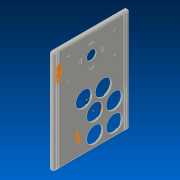
# Autodesk Inventor part: Top
Saved by Autodesk Inventor 2016 (Build 200138000, 138)
## iProperties
Created: 2015-08-21
Part Number: Top
Material: Generic
Document SubType Name: Modeling
Designer: Moffitt
Density: 1 g/cm^3
Appearance: Default
Author: Moffitt
Autodesk Inventor part; units mm, degrees
ref_plane "YZ Plane" through (0, 0, 0) normal (1, 0, 0) x (0, 1, 0)
ref_plane "XZ Plane" through (0, 0, 0) normal (0, 1, 0) x (-1, 0, 0)
ref_plane "XY Plane" through (0, 0, 0) normal (0, 0, 1) x (1, 0, 0)
sketch "Top-Body" plane through (0, 0, 0) normal (1, 0, 0) x (0, 1, 0)
  line L0 (107.2007, 64.0864) -> (-82.7993, 64.0864)
  line L1 (-82.7993, 64.0864) -> (-82.7993, -75.9136)
  line L2 (-82.7993, -75.9136) -> (107.2007, -75.9136)
  line L3 (107.2007, -75.9136) -> (107.2007, 64.0864)
  circle A0 centre (69.2007, -5.9136) radius 9
  circle A1 centre (6.2007, -27.9136) radius 15
  circle A2 centre (-24.2993, -47.9136) radius 15
  circle A3 centre (-60.2993, -47.9136) radius 15
  circle A4 centre (6.2007, 8.0864) radius 15
  circle A5 centre (-24.2993, -11.9136) radius 15
  circle A6 centre (-60.2993, -11.9136) radius 15
  circle A7 centre (89.2007, 36.0864) radius 2.5
  circle A8 centre (89.2007, -47.9136) radius 2.5
  circle A9 centre (49.2007, -47.9136) radius 2.5
  circle A10 centre (49.2007, 36.0864) radius 2.5
  point P0 (0, 0)
  dimension "d0" = 190
  dimension "d1" = 140
  dimension "d2" = 18
  dimension "d3" = 38
  dimension "d5" = 30
  dimension "d6" = 30
  dimension "d7" = 20
  dimension "d8" = 30.5
  dimension "d9" = 30
  dimension "d10" = 36
  dimension "d11" = 0
  dimension "d12" = 63
  dimension "d13" = 30
  dimension "d14" = 30
  dimension "d15" = 30
  dimension "d16" = 36
  dimension "d17" = 36
  dimension "d18" = 36
  dimension "d19" = 0
  dimension "d20" = 0
  dimension "d21" = 0
  dimension "d23" = 14
  dimension "d24" = 70
  dimension "d25" = 5
  dimension "d26" = 42
  dimension "d27" = 20
  dimension "d28" = 20
  dimension "d29" = 20
  dimension "d30" = 20
  dimension "d31" = 42
  dimension "d32" = 42
  dimension "d33" = 70
  dimension "d146" = 42
  dimension "d149" = 5
  dimension "d150" = 5
  dimension "d151" = 5
  constraints: 11 centre point, 8 end point, 2 parallel, 1 horizontal, 1 perpendicular
  measures "d0" distance of L0.start L0.end
  measures "d1" distance of L2.end L0.start
  measures "d2" diameter of A0
  measures "d3" distance from line of L3 A0.centre
  measures "d5" diameter of A1
  measures "d6" diameter of A2
  measures "d7" vertical distance of A2.centre A1.centre
  measures "d8" horizontal distance of A2.centre A1.centre
  measures "d9" diameter of A3
  measures "d10" distance of A3.centre A2.centre
  measures "d11" vertical distance of A3.centre A2.centre
  measures "d12" horizontal distance of A1.centre A0.centre
  measures "d13" diameter of A4
  measures "d14" diameter of A5
  measures "d15" diameter of A6
  measures "d16" distance of A1.centre A4.centre
  measures "d17" distance of A2.centre A5.centre
  measures "d18" distance of A3.centre A6.centre
  measures "d19" horizontal distance of A4.centre A1.centre
  measures "d20" horizontal distance of A5.centre A2.centre
  measures "d21" horizontal distance of A6.centre A3.centre
  measures "d23" vertical distance of A0.centre A4.centre
  measures "d24" distance from line of L2 A0.centre
  measures "d25" diameter of A7
  measures "d26" vertical distance of A0.centre A7.centre
  measures "d27" horizontal distance of A7.centre A0.centre
  measures "d28" horizontal distance of A10.centre A0.centre
  measures "d29" horizontal distance of A0.centre A8.centre
  measures "d30" horizontal distance of A9.centre A0.centre
  measures "d31" vertical distance of A0.centre A8.centre
  measures "d32" vertical distance of A9.centre A0.centre
  measures "d33" distance from line of L0 A0.centre
  measures "d146" vertical distance of A0.centre A10.centre
  measures "d149" diameter of A10
  measures "d150" diameter of A9
  measures "d151" diameter of A8
extrude "Main Face" add sketch "Top-Body" along normal blind 3
fillet "Top Fillet" radius 3 4 edges at (3, 107.2007, -5.9136) (3, 12.2007, 64.0864) (3, 12.2007, -75.9136) (3, -82.7993, -5.9136)
sketch "Button clip cutouts" plane through (0, 0, 0) normal (-1, 0, 0) x (0, 0, 1)
  line L0 (-33.0644, -51.1069) -> (-38.7212, -45.45)
  line L1 (-38.7212, -45.45) -> (-63.7628, -70.4917)
  line L2 (-63.7628, -70.4917) -> (-58.106, -76.1485)
  line L3 (-58.106, -76.1485) -> (-33.0644, -51.1069)
  line L4 (64.0864, -82.7993) -> (-75.9136, -82.7993) projected
  line L5 (3.9356, -70.4917) -> (-1.7212, -76.1485)
  line L6 (-1.7212, -76.1485) -> (-26.7628, -51.1069)
  line L7 (-26.7628, -51.1069) -> (-21.106, -45.45)
  line L8 (-21.106, -45.45) -> (3.9356, -70.4917)
  line L9 (-21.106, -39.1485) -> (-26.7628, -33.4917)
  line L10 (-26.7628, -33.4917) -> (-2.7212, -9.45)
  line L11 (-2.7212, -9.45) -> (2.9356, -15.1069)
  line L12 (2.9356, -15.1069) -> (-21.106, -39.1485)
  line L13 (-38.7212, -39.1485) -> (-33.0644, -33.4917)
  line L14 (-33.0644, -33.4917) -> (-57.106, -9.45)
  line L15 (-57.106, -9.45) -> (-62.7628, -15.1069)
  line L16 (-62.7628, -15.1069) -> (-38.7212, -39.1485)
  circle A0 centre (-47.9136, -24.2993) radius 15 projected
  circle A1 centre (-11.9136, -24.2993) radius 15 projected
  line L17 (-1.106, -8.6485) -> (-6.7628, -2.9917)
  line L18 (-6.7628, -2.9917) -> (17.2788, 21.05)
  line L19 (17.2788, 21.05) -> (22.9356, 15.3931)
  line L20 (22.9356, 15.3931) -> (-1.106, -8.6485)
  line L21 (-23.9136, -10.7993) -> (-31.9136, -10.7993)
  line L22 (-31.9136, -10.7993) -> (-31.9136, 23.2007)
  line L23 (-31.9136, 23.2007) -> (-23.9136, 23.2007)
  line L24 (-23.9136, 23.2007) -> (-23.9136, -10.7993)
  circle A2 centre (8.0864, 6.2007) radius 15 projected
  circle A3 centre (-27.9136, 6.2007) radius 15 projected
  circle A4 centre (-47.9136, -60.2993) radius 15 projected
  circle A5 centre (-11.9136, -60.2993) radius 15 projected
  point P0 (0, 0)
  dimension "d46" = 45
  dimension "d57" = 90
  dimension "d58" = 90
  dimension "d59" = 90
  dimension "d60" = 90
  dimension "d61" = 90
  dimension "d62" = 90
  dimension "d63" = 34
  dimension "d64" = 8
  dimension "d65" = 8
  dimension "d66" = 4
  dimension "d67" = 17
  dimension "d68" = 34
  dimension "d69" = 8
  dimension "d70" = 90
  dimension "d73" = 17
  dimension "d74" = 4
  dimension "d77" = 135
  dimension "d78" = 90
  dimension "d79" = 90
  dimension "d81" = 90
  dimension "d82" = 90
  dimension "d83" = 90
  dimension "d85" = 90
  dimension "d86" = 90
  dimension "d87" = 90
  dimension "d88" = 34
  dimension "d89" = 8
  dimension "d90" = 4
  dimension "d91" = 17
  dimension "d92" = 90
  dimension "d93" = 90
  dimension "d94" = 34
  dimension "d95" = 17
  dimension "d96" = 4
  dimension "d97" = 8
  dimension "d254" = 17
  dimension "d255" = 17
  dimension "d256" = 4
  dimension "d257" = 4
  dimension "d258" = 4
  dimension "d259" = 4
  constraints: 48 end point, 10 perpendicular, 1 horizontal, 1 parallel, 1 point on line
  measures "d46" angle of L4 L3
  measures "d57" angle of L10 L9
  measures "d58" angle of L11 L12
  measures "d59" angle of L9 L12
  measures "d60" angle of L10 L11
  measures "d61" angle of L16 L13
  measures "d62" angle of L15 L14
  measures "d63" distance between parallel lines of L15 L13
  measures "d64" distance of L13.start L13.end
  measures "d65" distance of L14.end L15.end
  measures "d66" distance from line of L14 A0.centre
  measures "d67" distance from line of L13 A0.centre
  measures "d68" distance of L9.end L10.end
  measures "d69" distance of L9.start L9.end
  measures "d70" angle of L14 L10
  measures "d73" distance from line of A1.centre L11
  measures "d74" distance from line of L10 A1.centre
  measures "d77" angle of L4 L8
  measures "d78" angle of L5 L8
  measures "d79" angle of L6 L7
  measures "d81" angle of L8 L12
  measures "d82" angle of L6 L3
  measures "d83" angle of L16 L1
  measures "d85" angle of L17 L20
  measures "d86" angle of L20 L19
  measures "d87" angle of L17 L10
  measures "d88" distance of L19.end L17.start
  measures "d89" distance of L18.end L19.end
  measures "d90" distance from line of L20 A2.centre
  measures "d91" distance from line of L17 A2.centre
  measures "d92" angle of L21 L24
  measures "d93" angle of L23 L22
  measures "d94" distance of L21.end L22.end
  measures "d95" distance from line of L21 A3.centre
  measures "d96" distance from line of L22 A3.centre
  measures "d97" distance of L22.end L23.end
  measures "d254" distance from line of L0 A4.centre
  measures "d255" distance from line of A5.centre L7
  measures "d256" distance from line of L8 A5.centre
  measures "d257" distance from line of A5.centre L6
  measures "d258" distance from line of L1 A4.centre
  measures "d259" distance from line of L3 A4.centre
extrude "Button Snap Cutouts" cut sketch "Button clip cutouts" against normal blind 1 contours L3 A4 L1 L0 | L3 A4 L1 | L3 L2 L1 A4 | L5 L6 A5 L8 | A5 L6 L8 | A5 L6 L7 L8 | L9 L10 A1 L12 | A1 L10 L12 | A1 L10 L11 L12 | L16 A0 L14 L13 | L16 A0 L14 | L16 L15 L14 A0 | L17 L18 A2 L20 | A2 L18 L20 | A2 L18 L19 L20 | L21 L22 A3 L24 | A3 L22 L24 | A3 L22 L23 L24
sketch "Insignias" plane through (3, 0, 0) normal (1, 0, 0) x (0, 0, -1)
  line L0 (24.9136, 74.2007) -> (24.9136, 64.2007)
  line L1 (24.9136, 64.2007) -> (29.9136, 69.2007)
  line L2 (29.9136, 69.2007) -> (24.9136, 74.2007)
  circle A0 centre (5.9136, 69.2007) radius 9 projected
  line L3 (10.9136, 50.2007) -> (0.9136, 50.2007)
  line L4 (0.9136, 50.2007) -> (5.9136, 45.2007)
  line L5 (5.9136, 45.2007) -> (10.9136, 50.2007)
  line L6 (10.9136, 87.2007) -> (0.9136, 87.2007)
  line L7 (0.9136, 87.2007) -> (5.9136, 92.2007)
  line L8 (5.9136, 92.2007) -> (10.9136, 87.2007)
  line L9 (-12.0864, 64.2007) -> (-12.0864, 74.2007)
  line L10 (-12.0864, 74.2007) -> (-17.0864, 69.2007)
  line L11 (-17.0864, 69.2007) -> (-12.0864, 64.2007)
  point P0 (0, 0)
  dimension "d117" = 45
  dimension "d118" = 45
  dimension "d119" = 10
  dimension "d120" = 10
  dimension "d121" = 5
  dimension "d122" = 45
  dimension "d123" = 45
  dimension "d124" = 10
  dimension "d125" = 10
  dimension "d126" = 5
  dimension "d127" = 19
  dimension "d128" = 18
  dimension "d129" = 18
  constraints: 24 end point, 3 perpendicular, 2 horizontal, 2 point on line, 1 vertical
  measures "d117" angle of L0 L2
  measures "d118" angle of L0 L1
  measures "d119" distance of L0.start L0.end
  measures "d120" distance edge to line of A0 L0
  measures "d121" vertical distance of A0.centre L0.start
  measures "d122" angle of L5 L3
  measures "d123" angle of L3 L4
  measures "d124" distance of L3.start L3.end
  measures "d125" distance edge to line of A0 L3
  measures "d126" horizontal distance of L3.end A0.centre
  measures "d127" distance from line of A0.centre L0
  measures "d128" distance from line of A0.centre L6
  measures "d129" distance from line of L9 A0.centre
extrude "Arrow signs" cut sketch "Insignias" against normal blind 0.5 contours L2 L1 L0 | L5 L4 L3 | L6 L7 L8 | L11 L10 L9
sketch "Sketch10" plane through (0, 0, 0) normal (-1, 0, 0) x (0, 0, 1)
  line L0 (-51.9136, 95.7007) -> (40.0864, 95.7007)
  line L1 (42.0864, 93.7007) -> (42.0864, 44.7007)
  line L2 (40.0864, 42.7007) -> (-51.9136, 42.7007)
  line L3 (-53.9136, 44.7007) -> (-53.9136, 93.7007)
  circle A0 centre (-47.9136, 89.2007) radius 2.5 projected
  circle A1 centre (-5.9136, 69.2007) radius 9 projected
  circle A2 centre (-47.9136, 49.2007) radius 2.5 projected
  arc A3 (-51.9136, 95.7007) -> (-53.9136, 93.7007) centre (-51.9136, 93.7007) ccw
  arc A4 (-53.9136, 44.7007) -> (-51.9136, 42.7007) centre (-51.9136, 44.7007) ccw
  arc A5 (40.0864, 42.7007) -> (42.0864, 44.7007) centre (40.0864, 44.7007) ccw
  arc A6 (42.0864, 93.7007) -> (40.0864, 95.7007) centre (40.0864, 93.7007) ccw
  point P0 (0, 0)
  point P1 (-53.9136, 95.7007)
  point P2 (42.0864, 95.7007)
  dimension "d155" = 96
  dimension "d157" = 48
  dimension "d158" = 6.5
  dimension "d159" = 6.5
  dimension "d160" = 2
  constraints: 8 end point, 8 point on circle, 8 tangent, 4 centre point, 4 point on line, 3 equal radius, 2 parallel, 1 horizontal, 1 perpendicular
  measures "d155" distance of point (-53.914, 95.701) point (42.086, 95.701)
  measures "d157" distance from line of L3 A1.centre
  measures "d158" vertical distance of point (-53.914, 95.701) A0.centre
  measures "d159" distance from line of L2 A2.centre
  measures "d160" radius of A3
extrude "JLF-P1 plate inset" cut sketch "Sketch10" against normal blind 1
sketch "Text" plane through (0, 0, 0) normal (-1, 0, 0) x (0, 0, 1)
  line L0 (53.0864, 77.2007) -> (52.0864, 77.2007)
  line L1 (52.0864, 77.2007) -> (52.0864, 76.2007)
  line L2 (52.0864, 76.2007) -> (49.0864, 76.2007)
  line L3 (49.0864, 76.2007) -> (49.0864, 77.2007)
  line L4 (49.0864, 77.2007) -> (50.0864, 77.2007)
  line L5 (50.0864, 77.2007) -> (50.0864, 78.2007)
  line L6 (50.0864, 78.2007) -> (48.0864, 78.2007)
  line L7 (48.0864, 78.2007) -> (48.0864, 75.2007)
  line L8 (48.0864, 75.2007) -> (52.0864, 75.2007)
  line L9 (52.0864, 75.2007) -> (52.0864, 74.2007)
  line L10 (52.0864, 74.2007) -> (53.0864, 74.2007)
  line L11 (53.0864, 74.2007) -> (53.0864, 77.2007)
  line L12 (53.0864, 73.2007) -> (48.0864, 73.2007)
  line L13 (48.0864, 73.2007) -> (48.0864, 69.2007)
  line L14 (48.0864, 69.2007) -> (49.0864, 69.2007)
  line L15 (49.0864, 69.2007) -> (49.0864, 72.2007)
  line L16 (49.0864, 72.2007) -> (53.0864, 72.2007)
  line L17 (53.0864, 72.2007) -> (53.0864, 73.2007)
  line L18 (53.0864, 68.2007) -> (53.0864, 65.2007)
  line L19 (53.0864, 65.2007) -> (52.0864, 65.2007)
  line L20 (52.0864, 65.2007) -> (52.0864, 67.2007)
  line L21 (52.0864, 67.2007) -> (51.0864, 67.2007)
  line L22 (51.0864, 67.2007) -> (51.0864, 66.2007)
  line L23 (51.0864, 66.2007) -> (50.0864, 66.2007)
  line L24 (50.0864, 66.2007) -> (50.0864, 67.2007)
  line L25 (53.0864, 68.2007) -> (48.0864, 68.2007)
  line L26 (48.0864, 68.2007) -> (48.0864, 67.2007)
  line L27 (48.0864, 67.2007) -> (50.0864, 67.2007)
  line L28 (51.0864, 64.2007) -> (50.0864, 64.2007)
  line L29 (50.0864, 64.2007) -> (50.0864, 62.2007)
  line L30 (50.0864, 62.2007) -> (51.0864, 62.2007)
  line L31 (51.0864, 62.2007) -> (51.0864, 64.2007)
  line L32 (48.0864, 61.2007) -> (53.0864, 61.2007)
  line L33 (53.0864, 61.2007) -> (53.0864, 59.2007)
  line L34 (53.0864, 59.2007) -> (52.0864, 59.2007)
  line L35 (52.0864, 59.2007) -> (52.0864, 60.2007)
  line L36 (52.0864, 60.2007) -> (51.0864, 60.2007)
  line L37 (51.0864, 60.2007) -> (51.0864, 59.2007)
  line L38 (51.0864, 59.2007) -> (50.0864, 59.2007)
  line L39 (50.0864, 59.2007) -> (50.0864, 60.2007)
  line L40 (50.0864, 60.2007) -> (48.0864, 60.2007)
  line L41 (48.0864, 60.2007) -> (48.0864, 61.2007)
  line L42 (52.0864, 59.2007) -> (51.0864, 59.2007)
  line L43 (51.0864, 58.2007) -> (52.0864, 58.2007)
  line L44 (52.0864, 58.2007) -> (52.0864, 59.2007)
  line L45 (51.0864, 59.2007) -> (51.0864, 58.2007)
  line L46 (52.0864, 57.2007) -> (51.0864, 57.2007)
  line L47 (51.0864, 57.2007) -> (51.0864, 56.2007)
  line L48 (51.0864, 56.2007) -> (52.0864, 56.2007)
  line L49 (52.0864, 56.2007) -> (52.0864, 57.2007)
  line L50 (53.0864, 56.2007) -> (48.0864, 56.2007)
  line L51 (48.0864, 56.2007) -> (48.0864, 55.2007)
  line L52 (48.0864, 55.2007) -> (53.0864, 55.2007)
  line L53 (53.0864, 55.2007) -> (53.0864, 56.2007)
  line L54 (18.0864, -47.7993) -> (13.0864, -47.7993)
  line L55 (13.0864, -47.7993) -> (13.0864, -49.7993)
  line L56 (13.0864, -49.7993) -> (14.0864, -49.7993)
  line L57 (14.0864, -49.7993) -> (14.0864, -50.7993)
  line L58 (14.0864, -50.7993) -> (15.0864, -50.7993)
  line L59 (15.0864, -50.7993) -> (15.0864, -49.7993)
  line L60 (15.0864, -49.7993) -> (16.0864, -49.7993)
  line L61 (16.0864, -49.7993) -> (16.0864, -50.7993)
  line L62 (16.0864, -50.7993) -> (17.0864, -50.7993)
  line L63 (17.0864, -50.7993) -> (17.0864, -49.7993)
  line L64 (17.0864, -49.7993) -> (18.0864, -49.7993)
  line L65 (18.0864, -49.7993) -> (18.0864, -47.7993)
  line L66 (17.0864, -49.7993) -> (16.0864, -49.7993)
  line L67 (16.0864, -49.7993) -> (16.0864, -48.7993)
  line L68 (16.0864, -48.7993) -> (17.0864, -48.7993)
  line L69 (17.0864, -48.7993) -> (17.0864, -49.7993)
  line L70 (15.0864, -49.7993) -> (14.0864, -49.7993)
  line L71 (14.0864, -49.7993) -> (14.0864, -48.7993)
  line L72 (14.0864, -48.7993) -> (15.0864, -48.7993)
  line L73 (15.0864, -48.7993) -> (15.0864, -49.7993)
  line L74 (14.0864, -51.7993) -> (13.0864, -51.7993)
  line L75 (13.0864, -51.7993) -> (13.0864, -54.7993)
  line L76 (13.0864, -54.7993) -> (14.0864, -54.7993)
  line L77 (14.0864, -54.7993) -> (16.0864, -54.7993)
  line L78 (16.0864, -54.7993) -> (16.0864, -52.7993)
  line L79 (16.0864, -52.7993) -> (17.0864, -52.7993)
  line L80 (17.0864, -52.7993) -> (17.0864, -54.7993)
  line L81 (17.0864, -54.7993) -> (18.0864, -54.7993)
  line L82 (18.0864, -54.7993) -> (18.0864, -51.7993)
  line L83 (18.0864, -51.7993) -> (15.0864, -51.7993)
  line L84 (15.0864, -51.7993) -> (15.0864, -53.7993)
  line L85 (15.0864, -53.7993) -> (14.0864, -53.7993)
  line L86 (14.0864, -53.7993) -> (14.0864, -51.7993)
  line L87 (13.0864, -55.7993) -> (18.0864, -55.7993)
  line L88 (18.0864, -55.7993) -> (18.0864, -58.7993)
  line L89 (18.0864, -58.7993) -> (17.0864, -58.7993)
  line L90 (17.0864, -58.7993) -> (17.0864, -56.7993)
  line L91 (17.0864, -56.7993) -> (16.0864, -56.7993)
  line L92 (16.0864, -56.7993) -> (16.0864, -57.7993)
  line L93 (16.0864, -57.7993) -> (15.0864, -57.7993)
  line L94 (15.0864, -57.7993) -> (15.0864, -56.7993)
  line L95 (15.0864, -56.7993) -> (13.0864, -56.7993)
  line L96 (13.0864, -56.7993) -> (13.0864, -55.7993)
  line L97 (60.0864, 103.2007) -> (-71.9136, 103.2007) projected
  arc A0 (-4.5195, -11.2483) -> (-24.9645, -31.6934) centre (-11.9136, -24.2993) ccw projected
  line L98 (18.0864, -46.7993) -> (13.0864, -46.7993)
  line L99 (13.0864, -46.7993) -> (13.0864, -43.7993)
  line L100 (13.0864, -43.7993) -> (18.0864, -43.7993)
  line L101 (18.0864, -43.7993) -> (18.0864, -46.7993)
  line L102 (17.0864, -44.7993) -> (14.0864, -44.7993)
  line L103 (14.0864, -44.7993) -> (14.0864, -45.7993)
  line L104 (14.0864, -45.7993) -> (17.0864, -45.7993)
  line L105 (17.0864, -45.7993) -> (17.0864, -44.7993)
  point P0 (0, 0)
  point P1 (1.3765, -19.3443)
  point P2 (-18.8686, -39.5894)
  dimension "d163" = 1
  dimension "d164" = 3
  dimension "d165" = 2
  dimension "d166" = 1
  dimension "d167" = 1
  dimension "d168" = 3
  dimension "d169" = 1
  dimension "d170" = 1
  dimension "d171" = 1
  dimension "d172" = 3
  dimension "d173" = 1
  dimension "d177" = 1
  dimension "d178" = 1
  dimension "d179" = 1
  dimension "d182" = 3
  dimension "d183" = 1
  dimension "d186" = 0
  dimension "d187" = 2
  dimension "d188" = 1
  dimension "d189" = 1
  dimension "d190" = 1
  dimension "d191" = 1
  dimension "d192" = 2
  dimension "d193" = 1
  dimension "d194" = 5
  dimension "d195" = 1
  dimension "d196" = 1
  dimension "d197" = 1
  dimension "d198" = 5
  dimension "d211" = 2
  dimension "d212" = 1
  dimension "d214" = 1
  dimension "d215" = 1
  dimension "d216" = 3
  dimension "d217" = 3
  dimension "d218" = 1
  dimension "d219" = 1
  dimension "d220" = 1
  dimension "d221" = 1
  dimension "d228" = 1
  dimension "d231" = 3
  dimension "d232" = 1
  dimension "d233" = 1
  dimension "d234" = 1
  dimension "d235" = 1
  constraints: 210 end point, 65 perpendicular, 41 point on line, 12 horizontal, 9 parallel, 1 vertical, 1 other
  measures "d163" distance of L0.start L0.end
  measures "d164" distance of L1.end L2.end
  measures "d165" distance of L5.end L6.end
  measures "d166" distance of L16.end L12.start
  measures "d167" distance between parallel lines of L2 L8
  measures "d168" distance of L10.end L0.start
  measures "d169" distance of L2.end L3.end
  measures "d170" distance of L4.end L5.end
  measures "d171" distance between parallel lines of L10 L12
  measures "d172" distance of L14.end L15.end
  measures "d173" distance of L13.end L14.end
  measures "d177" distance of L18.end L19.end
  measures "d178" distance of L20.end L21.end
  measures "d179" distance of L22.end L23.end
  measures "d182" distance of L18.start L18.end
  measures "d183" distance of L21.end L22.end
  measures "d186" distance between parallel lines of L18 L17
  measures "d187" distance of L30.end L28.start
  measures "d188" distance between parallel lines of L28 L19
  measures "d189" distance between parallel lines of L14 L25
  measures "d190" distance between parallel lines of L32 L30
  measures "d191" distance between parallel lines of L36 L32
  measures "d192" distance of L32.end L33.end
  measures "d193" distance of L37.end L43.start
  measures "d194" distance of L32.start L32.end
  measures "d195" distance of L48.end L46.start
  measures "d196" distance of L52.end L50.start
  measures "d197" distance between parallel lines of L43 L46
  measures "d198" distance of L51.end L52.end
  measures "d211" distance of L64.end L54.start
  measures "d212" distance of L62.end L63.end
  measures "d214" distance between parallel lines of L83 L62
  measures "d215" distance between parallel lines of L87 L81
  measures "d216" distance of L81.end L82.end
  measures "d217" distance of L87.end L88.end
  measures "d218" distance of L93.end L94.end
  measures "d219" distance of L95.end L87.start
  measures "d220" distance between parallel lines of L83 L79
  measures "d221" distance between parallel lines of L77 L85
  measures "d228" distance of L68.end L63.end
  measures "d231" distance of L100.end L98.start
  measures "d232" distance between parallel lines of L54 L98
  measures "d233" distance between parallel lines of L98 L104
  measures "d234" distance between parallel lines of L100 L102
  measures "d235" distance of L25.end L26.end
sketch "Sketch13" plane through (0, 0, 0) normal (-1, 0, 0) x (0, 0, 1)
  line L0 (64.0864, -82.7993) -> (-75.9136, -82.7993) projected
  line L1 (64.0864, 107.2007) -> (64.0864, -82.7993) projected
  line L2 (-75.9136, -82.7993) -> (64.0864, -82.7993)
  line L3 (64.0864, -82.7993) -> (64.0864, 107.2007)
  line L4 (64.0864, 107.2007) -> (-75.9136, 107.2007)
  line L5 (-75.9136, 107.2007) -> (-75.9136, -82.7993)
  line L6 (-74.4136, -81.2993) -> (62.5864, -81.2993)
  line L7 (62.5864, -81.2993) -> (62.5864, 105.7007)
  line L8 (62.5864, 105.7007) -> (-74.4136, 105.7007)
  line L9 (-74.4136, 105.7007) -> (-74.4136, -81.2993)
  point P0 (0, 0)
  dimension "d260" = 1.5
  dimension "d261" = 1.5
  dimension "d262" = 1.5
  dimension "d263" = 1.5
  constraints: 17 end point, 4 parallel, 2 horizontal, 2 perpendicular
  measures "d260" distance between parallel lines of L5 L9
  measures "d261" distance between parallel lines of L0 L6
  measures "d262" distance between parallel lines of L4 L8
  measures "d263" distance between parallel lines of L1 L7
extrude "Extrusion13" add sketch "Sketch13" along normal blind 3
fillet "Fillet4" radius 3 8 edges at (-1.5, -82.7993, 64.0864) (2.1213, -81.9206, 63.2078) (-1.5, -82.7993, -75.9136) (2.1213, -81.9206, -75.0349) (2.1213, 106.3221, -75.0349) (-1.5, 107.2007, -75.9136) (2.1213, 106.3221, 63.2078) (-1.5, 107.2007, 64.0864)
sketch "Sketch15" plane through (0, 0, 0) normal (-1, 0, 0) x (0, 0, 1)
  line L0 (61.0864, 104.2007) -> (-72.9136, 104.2007) projected
  line L1 (61.0864, 104.2007) -> (44.7033, 104.2007)
  line L2 (44.7033, 104.2007) -> (44.7033, 42.8326)
  line L3 (44.7033, 42.8326) -> (61.0864, 42.8326)
  line L4 (61.0864, 42.8326) -> (61.0864, 104.2007)
  line L5 (61.0864, -79.7993) -> (61.0864, 104.2007) projected
  line L6 (61.0864, 40.5103) -> (25.4802, 40.5103)
  line L7 (25.4802, 40.5103) -> (25.4802, -10.8372)
  line L8 (25.4802, -10.8372) -> (61.0864, -10.8372)
  line L9 (61.0864, -10.8372) -> (61.0864, 40.5103)
  line L10 (-72.9136, -79.7993) -> (61.0864, -79.7993) projected
  line L11 (61.0864, -13.6755) -> (7.1603, -13.6755)
  line L12 (7.1603, -13.6755) -> (7.1603, -79.7993)
  line L13 (7.1603, -79.7993) -> (61.0864, -79.7993)
  line L14 (61.0864, -79.7993) -> (61.0864, -13.6755)
  line L15 (22.6419, 40.5103) -> (-50.5089, 40.5103)
  line L16 (-50.5089, 40.5103) -> (-50.5089, 26.1898)
  line L17 (-50.5089, 26.1898) -> (22.6419, 26.1898)
  line L18 (22.6419, 26.1898) -> (22.6419, 40.5103)
  line L19 (-72.9136, 104.2007) -> (-72.9136, -79.7993) projected
  line L20 (-53.7342, 40.5103) -> (-72.9136, 40.5103)
  line L21 (-72.9136, 40.5103) -> (-72.9136, -6.8377)
  line L22 (-72.9136, -6.8377) -> (-53.7342, -6.8377)
  line L23 (-53.7342, -6.8377) -> (-53.7342, 40.5103)
  line L24 (-65.7325, -9.547) -> (-72.9136, -9.547)
  line L25 (-72.9136, -9.547) -> (-72.9136, -79.7993)
  line L26 (-72.9136, -79.7993) -> (-65.7325, -79.7993)
  line L27 (-65.7325, -79.7993) -> (-65.7325, -9.547)
  line L28 (-57.0886, 42.8326) -> (-72.9136, 42.8326)
  line L29 (-72.9136, 42.8326) -> (-72.9136, 101.5338)
  line L30 (-72.9136, 101.5338) -> (-57.0886, 101.5338)
  line L31 (-57.0886, 101.5338) -> (-57.0886, 42.8326)
  line L32 (-53.7342, 97.7924) -> (42.123, 97.7924)
  line L33 (42.123, 97.7924) -> (42.123, 104.2007)
  line L34 (42.123, 104.2007) -> (-53.7342, 104.2007)
  line L35 (-53.7342, 104.2007) -> (-53.7342, 97.7924)
  line L36 (-57.0886, 101.5338) -> (-72.9136, 101.5338)
  line L37 (-72.9136, 101.5338) -> (-72.9136, 104.2007)
  line L38 (-72.9136, 104.2007) -> (-57.0886, 104.2007)
  line L39 (-57.0886, 104.2007) -> (-57.0886, 101.5338)
  point P0 (0, 0)
  constraints: 72 end point, 18 parallel, 10 point on line, 9 horizontal, 9 perpendicular
extrude "Extrusion17" cut sketch "Sketch15" against normal blind 1 contours L4 L3 L2 L0 | L33 L32 L35 L0 | L5 L8 L7 L6 | L39 L30 L19 L0 | L5 L10 L12 L11 | L31 L28 L19 L30 | L10 L19 L24 L27 | L20 L23 L22 L19 | L18 L17 L16 L15
sketch "DMG lines" plane through (-3, 107.2007, 61.0864) normal (0, 1, 0) x (1, 0, 0)
  line L0 (6, 1.5) -> (4.5, 1.5)
  line L1 (4.5, 1.5) -> (4.5, 3.5)
  line L2 (4.5, 3.5) -> (6, 3.5)
  line L3 (6, 3.5) -> (6, 1.5)
  line L4 (6, 5.5) -> (4.5, 5.5)
  line L5 (4.5, 5.5) -> (4.5, 7.5)
  line L6 (4.5, 7.5) -> (6, 7.5)
  line L7 (6, 7.5) -> (6, 5.5)
  line L8 (6, 132.5) -> (4.5, 132.5)
  line L9 (4.5, 132.5) -> (4.5, 130.5)
  line L10 (4.5, 130.5) -> (6, 130.5)
  line L11 (6, 130.5) -> (6, 132.5)
  line L12 (6, 128.5) -> (4.5, 128.5)
  line L13 (4.5, 128.5) -> (4.5, 126.5)
  line L14 (4.5, 126.5) -> (6, 126.5)
  line L15 (6, 126.5) -> (6, 128.5)
  line L16 (3, 134) -> (3, 0) projected
  point P0 (3, 61.0864)
  point P1 (6, 134)
  point P2 (6, 0)
  dimension "d278" = 2
  dimension "d279" = 2
  dimension "d280" = 2
  dimension "d281" = 1.5
  dimension "d282" = 1.5
  dimension "d283" = 1.5
  dimension "d284" = 1.5
  dimension "d285" = 1.5
  dimension "d286" = 1.5
  dimension "d287" = 1.5
  dimension "d288" = 2
  dimension "d289" = 2
  dimension "d290" = 2
  dimension "d291" = 1.5
  dimension "d292" = 1.5
  constraints: 32 end point, 8 parallel, 4 horizontal, 4 perpendicular, 1 point on line
  measures "d278" distance between parallel lines of L10 L12
  measures "d279" distance of L12.end L13.end
  measures "d280" distance of L8.end L9.end
  measures "d281" distance from line of point (6, 134) L8
  measures "d282" distance of L13.end L14.end
  measures "d283" distance between parallel lines of L16 L13
  measures "d284" distance between parallel lines of L16 L9
  measures "d285" distance of L0.start L0.end
  measures "d286" distance of L4.start L4.end
  measures "d287" distance between parallel lines of L16 L1
  measures "d288" distance of L0.end L1.end
  measures "d289" distance between parallel lines of L4 L2
  measures "d290" distance of L4.end L5.end
  measures "d291" distance from line of point (6, 0) L0
  measures "d292" distance of L9.end L10.end
extrude "Extrusion19" cut sketch "DMG lines" against normal blind 190
body "Solid1"
